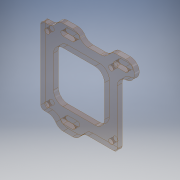
# Autodesk Inventor part: Pixy Bracket
Saved by Autodesk Inventor 2018 (Build 220112000, 112)
## iProperties
Created: 2018-08-30
Part Number: Pixy Bracket
Material: Polycarbonate, Smoke
Document SubType Name: Modeling
Designer: matth
Density: 1.2 g/cm^3
Appearance: Polycarbonate - Smoked
Author: matth
Autodesk Inventor part; units mm, degrees
ref_plane "YZ Plane" through (0, 0, 0) normal (1, 0, 0) x (0, 1, 0)
ref_plane "XZ Plane" through (0, 0, 0) normal (0, 1, 0) x (-1, 0, 0)
ref_plane "XY Plane" through (0, 0, 0) normal (0, 0, 1) x (1, 0, 0)
sketch "Sketch1" plane through (0, 0, 0) normal (0, 1, 0) x (-1, 0, 0)
  line L0 (0, 0) -> (0, -20)
  line L1 (0, -20) -> (-20, -20)
  line L2 (-20, -20) -> (-20, 20)
  line L3 (-20, 20) -> (20, 20)
  line L4 (20, 20) -> (20, -20)
  line L5 (20, -20) -> (0, -20)
  circle A0 centre (20, -20) radius 1.75
  circle A1 centre (-20, -20) radius 1.75
  circle A2 centre (-20, 20) radius 1.75
  circle A3 centre (20, 20) radius 1.75
  line L6 (20, -20) -> (20, -24)
  line L7 (20, -24) -> (24, -24)
  line L8 (24, -24) -> (16, -24)
  line L9 (16, -24) -> (16, 24)
  line L10 (16, 24) -> (24, 24)
  line L11 (24, 24) -> (24, -24)
  line L12 (16, 24) -> (-24, 24)
  line L13 (-24, 24) -> (-24, 16)
  line L14 (-24, 16) -> (16, 16)
  line L15 (16, 16) -> (16, 24)
  line L16 (-24, 16) -> (-16, 16)
  line L17 (-16, 16) -> (-16, -24)
  line L18 (-16, -24) -> (-24, -24)
  line L19 (-24, -24) -> (-24, 16)
  line L20 (-16, -24) -> (16, -24)
  line L21 (16, -24) -> (16, -16)
  line L22 (16, -16) -> (-16, -16)
  line L23 (-16, -16) -> (-16, -24)
  dimension "d0" = 20
  dimension "d1" = 20
  dimension "d2" = 40
  dimension "d3" = 40
  dimension "d4" = 40
  dimension "d5" = 3.5
  dimension "d6" = 3.5
  dimension "d7" = 3.5
  dimension "d8" = 3.5
  dimension "d9" = 4
  dimension "d10" = 4
  dimension "d11" = 8
  dimension "d12" = 48
  dimension "d13" = 40
  dimension "d14" = 8
  dimension "d15" = 8
  dimension "d16" = 40
  dimension "d17" = 8
  constraints: 48 end point, 8 parallel, 8 perpendicular, 4 centre point, 4 coincident, 4 horizontal, 2 point on line, 2 vertical
  measures "d0" distance of L0.start L0.end
  measures "d1" distance of L0.end L1.end
  measures "d2" distance of L1.end L2.end
  measures "d3" distance of L2.end L3.end
  measures "d4" distance of L3.end L4.end
  measures "d5" diameter of A0
  measures "d6" diameter of A1
  measures "d7" diameter of A2
  measures "d8" diameter of A3
  measures "d9" distance of L6.start L6.end
  measures "d10" distance of L6.end L7.end
  measures "d11" distance of L9.end L10.end
  measures "d12" distance of L8.end L9.end
  measures "d13" distance of L14.end L13.end
  measures "d14" distance of L13.end L12.end
  measures "d15" distance of L17.end L18.end
  measures "d16" distance of L16.end L17.end
  measures "d17" distance of L21.end L20.end
extrude "Extrusion1" add sketch "Sketch1" along normal blind 3 contours L22 L9 L5 L0 | L0 L1 L17 L22 | L5 L9 L20 L17 L1 | L17 L1 A1 L2 L14 | L17 L18 L19 L14 L2 A1 L1 | L14 L2 A2 L3 L9 | L3 A2 L2 L14 L13 L12 L9
sketch "Sketch2" plane through (0, 3, 0) normal (0, 1, 0) x (1, 0, 0)
  line L0 (-16, -24) -> (24, -24) projected
  line L1 (-16, -24) -> (-24, -24)
  line L2 (-24, -24) -> (-24, 24)
  line L3 (-24, 24) -> (-16, 24)
  line L4 (-16, 24) -> (-16, -24)
  circle A0 centre (-20, -20) radius 1.5
  circle A1 centre (-20, 20) radius 1.5
  circle A2 centre (20, -20) radius 1.75 projected
  circle A3 centre (20, -20) radius 1.75
  circle A4 centre (20, -20) radius 1.5
  circle A5 centre (20, 20) radius 1.75 projected
  circle A6 centre (20, 20) radius 1.75
  circle A7 centre (20, 20) radius 1.5
  point P0 (0, 0)
  dimension "d20" = 8
  dimension "d21" = 48
  dimension "d22" = 3
  dimension "d23" = 3
  dimension "d24" = 3
  dimension "d25" = 3
  constraints: 8 end point, 6 centre point, 4 coincident, 2 parallel, 1 horizontal, 1 perpendicular
  measures "d20" distance of L2.end L3.end
  measures "d21" distance of L1.end L2.end
  measures "d22" diameter of A0
  measures "d23" diameter of A1
  measures "d24" diameter of A4
  measures "d25" diameter of A7
extrude "Extrusion2" add sketch "Sketch2" against normal blind 3
fillet "Fillet1" radius 2 7 edges at (24, 1.5, 24) (-24, 1.5, 24) (-16, 1.5, 16) (16, 1.5, -16) (24, 1.5, -24) (-24, 1.5, -24) (-16, 1.5, -16)
fillet "Fillet3" radius 2 1 edges at (16, 1.5, 16)
sketch "Sketch6" plane through (0, 3, 0) normal (0, 1, 0) x (1, 0, 0)
  line L0 (0, 0) -> (-8.5, 0)
  line L1 (-8.5, 0) -> (-8.5, 15.33)
  line L2 (-8.5, 0) -> (-8.5, -15.33)
  line L3 (-8.5, -15.33) -> (24.5, -15.33)
  line L4 (-3.5, 15.33) -> (-13.5, 15.33) construction
  line L5 (-3.5, 17.08) -> (-13.5, 17.08)
  line L6 (-13.5, 13.58) -> (-3.5, 13.58)
  arc A0 (-3.5, 13.58) -> (-3.5, 17.08) centre (-3.5, 15.33) ccw
  arc A1 (-13.5, 17.08) -> (-13.5, 13.58) centre (-13.5, 15.33) ccw
  line L7 (-3.5, -15.33) -> (-13.5, -15.33) construction
  line L8 (-3.5, -13.58) -> (-13.5, -13.58)
  line L9 (-13.5, -17.08) -> (-3.5, -17.08)
  arc A2 (-3.5, -17.08) -> (-3.5, -13.58) centre (-3.5, -15.33) ccw
  arc A3 (-13.5, -13.58) -> (-13.5, -17.08) centre (-13.5, -15.33) ccw
  line L10 (29.5, -15.33) -> (19.5, -15.33) construction
  line L11 (29.5, -13.58) -> (19.5, -13.58)
  line L12 (19.5, -17.08) -> (29.5, -17.08)
  arc A4 (29.5, -17.08) -> (29.5, -13.58) centre (29.5, -15.33) ccw
  arc A5 (19.5, -13.58) -> (19.5, -17.08) centre (19.5, -15.33) ccw
  line L13 (29.5, -15.33) -> (19.5, -15.33) construction
  line L14 (29.5, -9.83) -> (19.5, -9.83)
  line L15 (19.5, -20.83) -> (29.5, -20.83)
  arc A6 (29.5, -20.83) -> (29.5, -9.83) centre (29.5, -15.33) ccw
  arc A7 (19.5, -9.83) -> (19.5, -20.83) centre (19.5, -15.33) ccw
  line L16 (-3.5, -15.33) -> (-13.5, -15.33) construction
  line L17 (-3.5, -9.83) -> (-13.5, -9.83)
  line L18 (-13.5, -20.83) -> (-3.5, -20.83)
  arc A8 (-3.5, -20.83) -> (-3.5, -9.83) centre (-3.5, -15.33) ccw
  arc A9 (-13.5, -9.83) -> (-13.5, -20.83) centre (-13.5, -15.33) ccw
  line L19 (-3.5, 15.33) -> (-13.5, 15.33) construction
  line L20 (-3.5, 20.83) -> (-13.5, 20.83)
  line L21 (-13.5, 9.83) -> (-3.5, 9.83)
  arc A10 (-3.5, 9.83) -> (-3.5, 20.83) centre (-3.5, 15.33) ccw
  arc A11 (-13.5, 20.83) -> (-13.5, 9.83) centre (-13.5, 15.33) ccw
  dimension "d54" = 8.5
  dimension "d55" = 15.33
  dimension "d56" = 15.33
  dimension "d57" = 33
  dimension "d58" = 5
  dimension "d59" = 3.5
  dimension "d60" = 5
  dimension "d61" = 3.5
  dimension "d62" = 5
  dimension "d63" = 3.5
  dimension "d64" = 11
  dimension "d65" = 11
  dimension "d66" = 11
  constraints: 56 end point, 24 point on circle, 24 tangent, 12 centre point, 6 midpoint, 6 parallel, 3 collinear, 2 horizontal, 2 perpendicular, 2 point on line, 1 vertical
  measures "d54" distance of L0.start L0.end
  measures "d55" distance of L0.end L1.end
  measures "d56" distance of L0.end L2.end
  measures "d57" distance of L2.end L3.end
  measures "d58" distance of L1.end L4.end
  measures "d59" diameter of A1
  measures "d60" distance of L2.end L7.end
  measures "d61" diameter of A3
  measures "d62" distance of L3.end L10.end
  measures "d63" diameter of A5
  measures "d64" diameter of A7
  measures "d65" diameter of A9
  measures "d66" diameter of A11
extrude "Extrusion6" add sketch "Sketch6" against normal blind 3 contours L17 A8 L3 A2 L8 L2 | L2 L8 A3 L9 A2 L3 A8 L18 A9 L17 | A6 L15 A7 L14 | A10 L21 A11 L20
sketch "Sketch7" plane through (0, 3, 0) normal (0, 1, 0) x (1, 0, 0)
  arc A0 (-3.5, 13.58) -> (-1.8833, 16) centre (-3.5, 15.33) ccw projected
  line L0 (-3.5, 15.33) -> (-8.5, 15.33)
  arc A1 (-1.8833, -16) -> (-3.5, -13.58) centre (-3.5, -15.33) ccw projected
  line L1 (-3.5, -15.33) -> (-8.5, -15.33)
  arc A2 (29.5, -17.08) -> (29.5, -13.58) centre (29.5, -15.33) ccw projected
  line L2 (29.5, -15.33) -> (24.5, -15.33)
  line L3 (-13.5, 15.33) -> (-3.5, 15.33) construction
  line L4 (-13.5, 17.08) -> (-3.5, 17.08)
  line L5 (-3.5, 13.58) -> (-13.5, 13.58)
  arc A3 (-13.5, 17.08) -> (-13.5, 13.58) centre (-13.5, 15.33) ccw
  arc A4 (-3.5, 13.58) -> (-3.5, 17.08) centre (-3.5, 15.33) ccw
  line L6 (-13.5, -15.33) -> (-3.5, -15.33) construction
  line L7 (-13.5, -17.08) -> (-3.5, -17.08)
  line L8 (-3.5, -13.58) -> (-13.5, -13.58)
  arc A5 (-13.5, -13.58) -> (-13.5, -17.08) centre (-13.5, -15.33) ccw
  arc A6 (-3.5, -17.08) -> (-3.5, -13.58) centre (-3.5, -15.33) ccw
  line L9 (19.5, -15.33) -> (29.5, -15.33) construction
  line L10 (19.5, -17.08) -> (29.5, -17.08)
  line L11 (29.5, -13.58) -> (19.5, -13.58)
  arc A7 (19.5, -13.58) -> (19.5, -17.08) centre (19.5, -15.33) ccw
  arc A8 (29.5, -17.08) -> (29.5, -13.58) centre (29.5, -15.33) ccw
  arc A9 (18.7149, -20.7737) -> (21.2494, -20.83) centre (20, -20) ccw projected
  circle A10 centre (20, -20) radius 1.5
  point P0 (0, 0)
  dimension "d69" = 5
  dimension "d70" = 5
  constraints: 30 end point, 12 point on circle, 12 tangent, 7 centre point, 3 collinear, 3 horizontal, 3 midpoint, 3 parallel, 2 concentric, 1 coincident
  measures "d69" distance of L0.start L0.end
  measures "d70" distance of L2.start L2.end
extrude "Extrusion7" cut sketch "Sketch7" against normal blind 3
fillet "Fillet4" radius 2 8 edges at (1.959, 1.5, -16) (-16, 1.5, -10.431) (-16, 1.5, 10.431) (1.959, 1.5, 16) (14.0409, 1.5, 15.9996) (16, 1.5, 11.0874) (24, 1.5, 20.83) (24, 1.5, 9.83)
sketch "Sketch9" plane through (0, 3, 0) normal (0, 1, 0) x (1, 0, 0)
  arc A0 (-13.5, -13.58) -> (-13.5, -17.08) centre (-13.5, -15.33) ccw projected
  arc A1 (-13.5, 17.08) -> (-13.5, 13.58) centre (-13.5, 15.33) ccw projected
  line L0 (12.1189, -16) -> (3.8811, -16) projected
  line L1 (-16, 7.8467) -> (-16, -7.8467) projected
  line L2 (7.0774, -16) -> (-16, -16)
  line L3 (-16, -16) -> (-16, -4.8403)
  line L4 (-16, -4.8403) -> (7.0774, -4.8403)
  line L5 (7.0774, -4.8403) -> (7.0774, -16)
  line L6 (-16, -16) -> (16, -16)
  line L7 (16, -16) -> (16, 16)
  line L8 (16, 16) -> (-16, 16)
  line L9 (-16, 16) -> (-16, -16)
  point P0 (0, 0)
  dimension "d82" = 32
  constraints: 16 end point, 4 parallel, 2 horizontal, 2 perpendicular, 2 point on line
  measures "d82" distance of L8.end L7.end
extrude "Extrusion9" cut sketch "Sketch9" against normal blind 10
sketch "Sketch10" plane through (0, 3, 0) normal (0, 1, 0) x (1, 0, 0)
  line L0 (24, -7.83) -> (24, 22) projected
  line L1 (24, 1.8484) -> (40.3961, 1.8484)
  line L2 (40.3961, 1.8484) -> (40.3961, -29.4737)
  line L3 (40.3961, -29.4737) -> (24, -29.4737)
  line L4 (24, -29.4737) -> (24, 1.8484)
  point P0 (0, 0)
  constraints: 8 end point, 2 parallel, 1 horizontal, 1 perpendicular, 1 point on line
extrude "Extrusion10" cut sketch "Sketch10" against normal blind 10
sketch "Sketch11" plane through (0, 3, 0) normal (0, 1, 0) x (1, 0, 0)
  line L0 (24, -17.08) -> (24, -22.2463) projected
  line L1 (16, 16) -> (16, -16) projected
  line L2 (24, -18.1637) -> (16, -18.1637)
  line L3 (16, -18.1637) -> (16, -10.7114)
  line L4 (16, -10.7114) -> (24, -10.7114)
  line L5 (24, -10.7114) -> (24, -18.1637)
  line L6 (16, -16) -> (-1.8833, -16) projected
  line L7 (6.5639, -16) -> (-15.8817, -16)
  line L8 (-15.8817, -16) -> (-15.8817, -19.7163)
  line L9 (-15.8817, -19.7163) -> (6.5639, -19.7163)
  line L10 (6.5639, -19.7163) -> (6.5639, -16)
  line L11 (-1.8833, 16) -> (16, 16) projected
  line L12 (2.0393, 16) -> (-16.9463, 16)
  line L13 (-16.9463, 16) -> (-16.9463, 18.0775)
  line L14 (-16.9463, 18.0775) -> (2.0393, 18.0775)
  line L15 (2.0393, 18.0775) -> (2.0393, 16)
  point P0 (0, 0)
  constraints: 24 end point, 6 parallel, 4 point on line, 3 horizontal, 3 perpendicular
extrude "Extrusion11" add sketch "Sketch11" against normal blind 3
sketch "Sketch12" plane through (0, 3, 0) normal (0, 1, 0) x (1, 0, 0)
  line L0 (0, 0) -> (-6.92, 0)
  line L1 (-6.92, 0) -> (-6.92, -23.8)
  line L2 (-3.92, -23.8) -> (-9.92, -23.8) construction
  line L3 (-3.92, -22.3) -> (-9.92, -22.3)
  line L4 (-9.92, -25.3) -> (-3.92, -25.3)
  arc A0 (-3.92, -25.3) -> (-3.92, -22.3) centre (-3.92, -23.8) ccw
  arc A1 (-9.92, -22.3) -> (-9.92, -25.3) centre (-9.92, -23.8) ccw
  line L5 (-6.92, 0) -> (-6.92, 23.8)
  line L6 (-9.92, 23.8) -> (-3.92, 23.8) construction
  line L7 (22, 24) -> (-22, 24) projected
  line L8 (-9.92, 22.3) -> (-3.92, 22.3)
  line L9 (-3.92, 25.3) -> (-9.92, 25.3)
  arc A2 (-9.92, 25.3) -> (-9.92, 22.3) centre (-9.92, 23.8) ccw
  arc A3 (-3.92, 22.3) -> (-3.92, 25.3) centre (-3.92, 23.8) ccw
  line L10 (-6.92, 23.8) -> (-0.92, 23.8) construction
  line L11 (-9.92, 23.8) -> (-3.92, 23.8) construction
  line L12 (-9.92, 18.3) -> (-3.92, 18.3)
  line L13 (-3.92, 29.3) -> (-9.92, 29.3)
  arc A4 (-9.92, 29.3) -> (-9.92, 18.3) centre (-9.92, 23.8) ccw
  arc A5 (-3.92, 18.3) -> (-3.92, 29.3) centre (-3.92, 23.8) ccw
  line L14 (-3.92, -23.8) -> (-9.92, -23.8) construction
  line L15 (-3.92, -18.3) -> (-9.92, -18.3)
  line L16 (-9.92, -29.3) -> (-3.92, -29.3)
  arc A6 (-3.92, -29.3) -> (-3.92, -18.3) centre (-3.92, -23.8) ccw
  arc A7 (-9.92, -18.3) -> (-9.92, -29.3) centre (-9.92, -23.8) ccw
  line L17 (-6.92, -23.8) -> (26.28, -23.8)
  line L18 (-6.92, -23.8) -> (26.28, -23.8) construction
  line L19 (23.28, -23.8) -> (29.28, -23.8) construction
  line L20 (23.28, -25.3) -> (29.28, -25.3)
  line L21 (29.28, -22.3) -> (23.28, -22.3)
  arc A8 (23.28, -22.3) -> (23.28, -25.3) centre (23.28, -23.8) ccw
  arc A9 (29.28, -25.3) -> (29.28, -22.3) centre (29.28, -23.8) ccw
  line L22 (23.28, -23.8) -> (29.28, -23.8) construction
  line L23 (23.28, -29.3) -> (29.28, -29.3)
  line L24 (29.28, -18.3) -> (23.28, -18.3)
  arc A10 (23.28, -18.3) -> (23.28, -29.3) centre (23.28, -23.8) ccw
  arc A11 (29.28, -29.3) -> (29.28, -18.3) centre (29.28, -23.8) ccw
  dimension "d89" = 6.92
  dimension "d90" = 23.8
  dimension "d91" = 3
  dimension "d92" = 3
  dimension "d93" = 23.8
  dimension "d94" = 3
  dimension "d95" = 0
  dimension "d96" = 3
  dimension "d97" = 11
  dimension "d98" = 11
  dimension "d99" = 33.2
  dimension "d100" = 0
  dimension "d101" = 3
  dimension "d102" = 3
  dimension "d103" = 11
  constraints: 60 end point, 24 point on circle, 24 tangent, 12 centre point, 10 parallel, 6 horizontal, 6 midpoint, 2 collinear, 2 vertical
  measures "d89" distance of L0.start L0.end
  measures "d90" distance of L0.end L1.end
  measures "d91" distance of L1.end L2.end
  measures "d92" diameter of A1
  measures "d93" distance of L0.end L5.end
  measures "d94" distance of L5.end L6.end
  measures "d95" distance between parallel lines of L6 L10
  measures "d96" diameter of A3
  measures "d97" diameter of A5
  measures "d98" diameter of A7
  measures "d99" distance of L1.end L17.end
  measures "d100" distance between parallel lines of L17 L18
  measures "d101" distance of L18.end L19.end
  measures "d102" diameter of A9
  measures "d103" diameter of A11
extrude "Extrusion12" add sketch "Sketch12" against normal blind 3 contours L15 A6 L17 A0 L3 L1 | L1 L3 A1 L4 A0 L17 A6 L16 A7 L15 | L12 A4 L7 A2 L8 L5 | L5 L8 A3 L7 A5 L12 | A4 L13 A5 L7 A3 L9 A2 | A10 L24 A11 L23
sketch "Sketch13" plane through (0, 3, 0) normal (0, 1, 0) x (1, 0, 0)
  arc A0 (29.28, -25.3) -> (29.28, -22.3) centre (29.28, -23.8) ccw projected
  line L0 (29.28, -23.8) -> (26.28, -23.8)
  arc A1 (-3.92, -25.3) -> (-2.4334, -24) centre (-3.92, -23.8) ccw projected
  line L1 (-3.92, -23.8) -> (-6.92, -23.8)
  arc A2 (-2.4334, 24) -> (-3.92, 25.3) centre (-3.92, 23.8) ccw projected
  line L2 (-3.92, 23.8) -> (-6.92, 23.8)
  line L3 (-9.92, 23.8) -> (-3.92, 23.8) construction
  line L4 (-9.92, 22.3) -> (-3.92, 22.3)
  line L5 (-3.92, 25.3) -> (-9.92, 25.3)
  arc A3 (-9.92, 25.3) -> (-9.92, 22.3) centre (-9.92, 23.8) ccw
  arc A4 (-3.92, 22.3) -> (-3.92, 25.3) centre (-3.92, 23.8) ccw
  line L6 (-9.92, -23.8) -> (-3.92, -23.8) construction
  line L7 (-9.92, -25.3) -> (-3.92, -25.3)
  line L8 (-3.92, -22.3) -> (-9.92, -22.3)
  arc A5 (-9.92, -22.3) -> (-9.92, -25.3) centre (-9.92, -23.8) ccw
  arc A6 (-3.92, -25.3) -> (-3.92, -22.3) centre (-3.92, -23.8) ccw
  line L9 (23.28, -23.8) -> (29.28, -23.8) construction
  line L10 (23.28, -25.3) -> (29.28, -25.3)
  line L11 (29.28, -22.3) -> (23.28, -22.3)
  arc A7 (23.28, -22.3) -> (23.28, -25.3) centre (23.28, -23.8) ccw
  arc A8 (29.28, -25.3) -> (29.28, -22.3) centre (29.28, -23.8) ccw
  arc A9 (20.9333, -18.8257) -> (18.702, -20.7518) centre (20, -20) ccw projected
  circle A10 centre (20, -20) radius 1.5
  point P0 (0, 0)
  dimension "d106" = 3
  dimension "d107" = 3
  dimension "d108" = 3
  constraints: 30 end point, 12 point on circle, 12 tangent, 7 centre point, 3 collinear, 3 concentric, 3 horizontal, 3 midpoint, 3 parallel, 1 coincident
  measures "d106" distance of L0.start L0.end
  measures "d107" distance of L1.start L1.end
  measures "d108" distance of L2.start L2.end
extrude "Extrusion13" cut sketch "Sketch13" against normal blind 3
fillet "Fillet5" radius 6 10 edges at (17.7836, 1.5, 24) (1.5764, 1.5, 24) (-15.4164, 1.5, 24) (-15.4164, 1.5, -24) (1.5764, 1.5, -24) (24, 1.5, 18.3) (16, 1.5, 16) (-16, 1.5, 16) (-16, 1.5, -16) (16, 1.5, -16)
body "Solid1"
